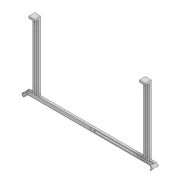
# Autodesk Inventor part: Bancada
Saved by Autodesk Inventor 2021 (Build 250183000, 183)
## iProperties
Created: 2021-04-19
Part Number: Bancada
Material: Genérico
Document SubType Name: Modeling
Designer: carlo
Density: 1 g/cm^3
Appearance: Valor por defecto
Author: carlo
Autodesk Inventor part; units mm, degrees
ref_plane "YZ Plane" through (0, 0, 0) normal (1, 0, 0) x (0, 1, 0)
ref_plane "XZ Plane" through (0, 0, 0) normal (0, 1, 0) x (-1, 0, 0)
ref_plane "XY Plane" through (0, 0, 0) normal (0, 0, 1) x (1, 0, 0)
sketch "Boceto1" plane through (0, 0, 0) normal (0, 0, 1) x (1, 0, 0)
  arc A0 (160, -5) -> (160, 5) centre (160, 0) ccw
  arc A1 (160, -2.5) -> (160, 2.5) centre (160, 0) ccw
  circle A2 centre (0, 0) radius 2.5
  line L0 (0, -5) -> (160, -5)
  line L1 (160, -2.5) -> (8, -2.5)
  line L2 (8, -2.5) -> (8, 2.5)
  line L3 (8, 2.5) -> (160, 2.5)
  line L4 (160, 2.5) -> (160, -2.5)
  line L5 (140, 5) -> (142.5, 5)
  line L6 (142.5, 5) -> (137.5, 5)
  line L7 (137.5, 5) -> (137.5, 174)
  line L8 (142.5, 174) -> (142.5, 5)
  line L9 (132.5, 179) -> (147.5, 179)
  line L10 (147.5, 179) -> (147.5, 5)
  line L11 (142.5, 5) -> (137.5, 5)
  line L12 (132.5, 5) -> (132.5, 179)
  line L13 (137.5, 174) -> (142.5, 174)
  line L14 (147.5, 5) -> (160, 5)
  line L15 (0, 5) -> (132.5, 5)
  line L16 (137.5, 5) -> (142.5, 5)
  line L17 (0, -2.5) -> (0, 2.5)
  arc A3 (-160, 5) -> (-160, -5) centre (-160, 0) ccw
  line L18 (0, -5) -> (-160, -5)
  line L19 (-140, 5) -> (-142.5, 5)
  line L20 (-142.5, 5) -> (-137.5, 5)
  line L21 (-137.5, 5) -> (-137.5, 174)
  line L22 (-142.5, 174) -> (-142.5, 5)
  line L23 (-132.5, 179) -> (-147.5, 179)
  line L24 (-147.5, 179) -> (-147.5, 5)
  line L25 (-142.5, 5) -> (-137.5, 5)
  line L26 (-132.5, 5) -> (-132.5, 179)
  line L27 (-137.5, 174) -> (-142.5, 174)
  line L28 (-147.5, 5) -> (-160, 5)
  line L29 (0, 5) -> (-132.5, 5)
  line L30 (-137.5, 5) -> (-142.5, 5)
  dimension "d2" = 10
  dimension "d3" = 5
  dimension "d4" = 5
  dimension "d13" = 15
  dimension "d17" = 174
  dimension "d18" = 169
  constraints: 62 end point, 12 symmetric about line, 8 parallel, 8 point on circle, 4 centre point, 4 perpendicular, 3 horizontal, 3 tangent, 1 coincident, 1 vertical, 1 other
  measures "d2" diameter of A0
  measures "d3" diameter of A1
  measures "d4" diameter of A2
  measures "d13" distance of L10.end L12.start
  measures "d17" distance of L12.start L9.start
  measures "d18" distance between parallel lines of L15 L13
extrude "Extrusión1" add sketch "Boceto1" along normal blind 5
sketch "Boceto3" plane through (0, 0, 5) normal (0, 0, 1) x (1, 0, 0)
  circle A0 centre (0, 0) radius 2.5 projected
  arc A1 (-160, 5) -> (-160, -5) centre (-160, 0) ccw
  arc A2 (-160, 5) -> (-160, -5) centre (-160, 0) ccw projected
  line L0 (-160, -5) -> (160, -5) projected
  arc A3 (-160, 2.5) -> (-160, -2.5) centre (-160, 0) ccw
  line L1 (-160, 2.5) -> (-160, 5)
  line L2 (-160, -2.5) -> (-160, -5)
  circle A4 centre (0, 0) radius 2.5 projected
  line L3 (8, 2.5) -> (160, 2.5) projected
  arc A5 (160, -5) -> (160, 5) centre (160, 0) ccw
  arc A6 (160, -2.5) -> (160, 2.5) centre (160, 0) ccw
  arc A7 (160, -5) -> (160, 5) centre (160, 0) ccw projected
  line L4 (160, -5) -> (160, -2.5)
  line L5 (160, 2.5) -> (160, 5)
  line L6 (-132.5, 179) -> (-147.5, 179) projected
  line L7 (-147.5, 179) -> (-132.5, 179)
  line L8 (-132.5, 179) -> (-132.5, 174)
  line L9 (-132.5, 174) -> (-147.5, 174)
  line L10 (-147.5, 174) -> (-147.5, 179)
  line L11 (147.5, 5) -> (147.5, 179) projected
  line L12 (132.5, 179) -> (147.5, 179)
  line L13 (147.5, 179) -> (147.5, 174)
  line L14 (147.5, 174) -> (132.5, 174)
  line L15 (132.5, 174) -> (132.5, 179)
  dimension "d23" = 5
  dimension "d24" = 15
  dimension "d25" = 5
  constraints: 25 end point, 8 point on circle, 5 equal length, 4 centre point, 3 coincident, 3 vertical, 2 horizontal, 2 perpendicular, 1 point on line, 2 other
  measures "d23" diameter of A3
  measures "d24" distance of L8.end L9.end
  measures "d25" distance of L7.end L8.end
extrude "Extrusión2" add sketch "Boceto3" along normal blind 10 contours L1 A3 L2 A1 | L4 A6 L5 A5 | L8 L9 L10 L6 | L14 L15 L12 L11
